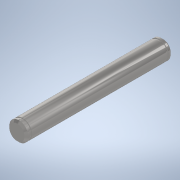
# Autodesk Inventor part: SHAFT
Saved by Autodesk Inventor 2022 (Build 260153000, 153)
## iProperties
Created: 2022-07-25
Part Number: SHAFT
Material: Stainless Steel
Document SubType Name: Modeling
Designer: Nathan Cai
Density: 8 g/cm^3
Appearance: Semi-Polished
Author: Nathan Cai
Autodesk Inventor part; units mm, degrees
ref_plane "YZ Plane" through (0, 0, 0) normal (1, 0, 0) x (0, 1, 0)
ref_plane "XZ Plane" through (0, 0, 0) normal (0, 1, 0) x (-1, 0, 0)
ref_plane "XY Plane" through (0, 0, 0) normal (0, 0, 1) x (1, 0, 0)
sketch "Sketch1" plane through (0, 0, 0) normal (0, 1, 0) x (-1, 0, 0)
  line L0 (0, 0) -> (2.5, 0)
  line L1 (2.5, 0) -> (2.5, -38.5)
  line L2 (2.5, -38.5) -> (0, -38.5)
  line L3 (0, -38.5) -> (0, 0)
  line L4 (2.5, -37.5) -> (2.25, -37.5)
  line L5 (2.25, -37.5) -> (2.25, -37)
  line L6 (2.25, -37) -> (2.5, -37)
  line L7 (2.5, -37) -> (2.5, -37.5)
  line L8 (2.5, -19.25) -> (0, -19.25) construction
  line L9 (2.5, -1) -> (2.25, -1)
  line L10 (2.25, -1) -> (2.25, -1.5)
  line L11 (2.25, -1.5) -> (2.5, -1.5)
  line L12 (2.5, -1.5) -> (2.5, -1)
  dimension "d0" = 2.5
  dimension "d1" = 38.5
  dimension "d2" = 0.25
  dimension "d3" = 0.5
  dimension "d4" = 1
  constraints: 26 end point, 4 parallel, 4 symmetric about line, 2 horizontal, 2 midpoint, 2 perpendicular, 1 point on line
  measures "d0" distance of L1.end L2.end
  measures "d1" distance of L0.end L1.end
  measures "d2" distance of L5.end L6.end
  measures "d3" distance of L4.end L5.end
  measures "d4" distance between parallel lines of L2 L4
revolve "Revolution1" add sketch "Sketch1" angle 360 about axis through (0, 0, -38.5) along (0, 0, 1) contours L0 L1 L9 L10 L11 L6 L5 L4 L2 L3
chamfer "Chamfer1" distance 0.5 angle 45 2 edges at (2.5, 0, 0) (2.5, 0, -38.5)
body "Solid1"
